Autodesk Fusion 360 part; units mm, degrees
note: some values were not read from the file. Set by a fixed rule: which sketch regions a step uses.
(part 4 of 14)
  spline S16 degree 5 poles (-6.8027, -18.1294) (-6.8027, -18.1295) (-6.8028, -18.1296) (-6.8029, -18.1298) (-6.803, -18.1302) (-6.8032, -18.1308) (-6.8035, -18.1315) (-6.8037, -18.1322) (-6.804, -18.133) (-6.8043, -18.1339) (-6.8047, -18.1349) (-6.8051, -18.136) (-6.8055, -18.1372) (-6.8059, -18.1384) (-6.8063, -18.1397) (-6.8068, -18.1411) (-6.8073, -18.1426) (-6.8078, -18.1442) (-6.8083, -18.1458) (-6.8089, -18.1475) (-6.8095, -18.1493) (-6.8101, -18.1512) (-6.8107, -18.1531) (-6.8113, -18.1552) (-6.812, -18.1572) (-6.8127, -18.1594) (-6.8134, -18.1617) (-6.8141, -18.164) (-6.8148, -18.1663) (-6.8155, -18.1688) (-6.8163, -18.1713) (-6.8171, -18.1739) (-6.8179, -18.1766) (-6.8187, -18.1793) (-6.8195, -18.1821) (-6.8203, -18.185) (-6.8212, -18.1879) (-6.822, -18.191) (-6.8229, -18.194) (-6.8238, -18.1972) (-6.8247, -18.2004) (-6.8256, -18.2037) (-6.8265, -18.207) (-6.8274, -18.2104) (-6.8284, -18.2139) (-6.8293, -18.2174) (-6.8303, -18.221) (-6.8312, -18.2247) (-6.8322, -18.2284) (-6.8332, -18.2322) (-6.8342, -18.236) (-6.8352, -18.2399) (-6.8362, -18.2439) (-6.8372, -18.2479) (-6.8382, -18.252) (-6.8392, -18.2561) (-6.8403, -18.2604) (-6.8413, -18.2646) (-6.8424, -18.269) (-6.8434, -18.2733) (-6.8445, -18.2778) (-6.8455, -18.2823) (-6.8466, -18.2868) (-6.8477, -18.2915) (-6.8487, -18.2961) (-6.8498, -18.3009) (-6.8509, -18.3057) (-6.852, -18.3105) (-6.8531, -18.3154) (-6.8542, -18.3203) (-6.8553, -18.3254) (-6.8564, -18.3304) (-6.8575, -18.3355) (-6.8586, -18.3407) (-6.8597, -18.3459) (-6.8608, -18.3512) (-6.8619, -18.3565) (-6.863, -18.3619) (-6.8641, -18.3674) (-6.8652, -18.3729) (-6.8663, -18.3784) (-6.8674, -18.384) (-6.8685, -18.3896) (-6.8696, -18.3953) (-6.8707, -18.4011) (-6.8718, -18.4069) (-6.8729, -18.4127) (-6.874, -18.4186) (-6.8751, -18.4246) (-6.8762, -18.4306) (-6.8773, -18.4366) (-6.8784, -18.4427) (-6.8795, -18.4489) (-6.8805, -18.4551) (-6.8816, -18.4613) (-6.8827, -18.4676) (-6.8838, -18.474) (-6.8849, -18.4804) (-6.8859, -18.4868) (-6.887, -18.4933) (-6.8881, -18.4998) (-6.8891, -18.5064) (-6.8902, -18.513) (-6.8912, -18.5197) (-6.8923, -18.5264) (-6.8933, -18.5332) (-6.8944, -18.54) (-6.8954, -18.5469) (-6.8964, -18.5538) (-6.8974, -18.5607) (-6.8985, -18.5677) (-6.8995, -18.5747) (-6.9005, -18.5818) (-6.9015, -18.5889) (-6.9025, -18.5961) (-6.9034, -18.6033) (-6.9044, -18.6106) (-6.9054, -18.6179) (-6.9064, -18.6252) (-6.9073, -18.6326) (-6.9083, -18.6401) (-6.9092, -18.6475) (-6.9102, -18.6551) (-6.9111, -18.6626) (-6.912, -18.6702) (-6.9129, -18.6779) (-6.9138, -18.6856) (-6.9147, -18.6933) (-6.9156, -18.7011) (-6.9165, -18.7089) (-6.9174, -18.7167) (-6.9182, -18.7246) (-6.9191, -18.7326) (-6.9199, -18.7405) (-6.9208, -18.7485) (-6.9216, -18.7566) (-6.9224, -18.7647) (-6.9232, -18.7728) (-6.924, -18.781) (-6.9248, -18.7892) (-6.9256, -18.7975) (-6.9264, -18.8058) (-6.9272, -18.8141) (-6.9279, -18.8225) (-6.9287, -18.8309) (-6.9294, -18.8394) (-6.9301, -18.8479) (-6.9308, -18.8564) (-6.9315, -18.8649) (-6.9322, -18.8736) (-6.9329, -18.8822) (-6.9336, -18.8909) (-6.9342, -18.8996) (-6.9349, -18.9084) (-6.9355, -18.9171) (-6.9361, -18.926) (-6.9367, -18.9348) (-6.9373, -18.9438) (-6.9379, -18.9527) (-6.9385, -18.9617) (-6.9391, -18.9707) (-6.9396, -18.9797) (-6.9402, -18.9888) (-6.9407, -18.9979) (-6.9412, -19.0071) (-6.9417, -19.0163) (-6.9422, -19.0255) (-6.9427, -19.0348) (-6.9431, -19.0441) (-6.9436, -19.0534) (-6.944, -19.0628) (-6.9445, -19.0722) (-6.9449, -19.0816) (-6.9453, -19.0911) (-6.9457, -19.1006) (-6.946, -19.1102) (-6.9464, -19.1198) (-6.9467, -19.1294) (-6.9471, -19.139) (-6.9474, -19.1487) (-6.9477, -19.1584) (-6.948, -19.1681) (-6.9483, -19.1779) (-6.9485, -19.1877) (-6.9488, -19.1976) (-6.949, -19.2075) (-6.9492, -19.2174) (-6.9495, -19.2273) (-6.9496, -19.2373) (-6.9498, -19.2473) (-6.95, -19.2574) (-6.9501, -19.2674) (-6.9503, -19.2775) (-6.9504, -19.2877) (-6.9505, -19.2979) (-6.9506, -19.3081) (-6.9507, -19.3183) (-6.9507, -19.3286) (-6.9508, -19.3389) (-6.9508, -19.3492) (-6.9508, -19.3595) (-6.9508, -19.3699) (-6.9508, -19.3804) (-6.9507, -19.3908) (-6.9507, -19.4013) (-6.9506, -19.4118) (-6.9505, -19.4224) (-6.9505, -19.4329) (-6.9503, -19.4435) (-6.9502, -19.4542) (-6.9501, -19.4648) (-6.9499, -19.4755) (-6.9497, -19.4863) (-6.9495, -19.497) (-6.9493, -19.5078) (-6.9491, -19.5186) (-6.9488, -19.5295) (-6.9486, -19.5403) (-6.9483, -19.5512) (-6.948, -19.5622) (-6.9477, -19.5731) (-6.9474, -19.5841) (-6.947, -19.5951) (-6.9467, -19.6062) (-6.9463, -19.6172) (-6.9459, -19.6283) (-6.9455, -19.6395) (-6.9451, -19.6506) (-6.9446, -19.6618) (-6.9441, -19.673) (-6.9437, -19.6843) (-6.9432, -19.6956) (-6.9426, -19.7068) (-6.9421, -19.7182) (-6.9416, -19.7295) (-6.941, -19.7409) (-6.9404, -19.7523) (-6.9398, -19.7637) (-6.9392, -19.7752) (-6.9385, -19.7867) (-6.9379, -19.7982) (-6.9373, -19.8074) (-6.9369, -19.8144) (-6.9366, -19.819) (-6.9365, -19.8213) knots 0 0 0 0 0 0 0.00416667 0.00833333 0.0125 0.01666667 0.02083333 0.025 0.02916667 0.03333333 0.0375 0.04166667 0.04583333 0.05 0.05416667 0.05833333 0.0625 0.06666667 0.07083333 0.075 0.07916667 0.08333333 0.0875 0.09166667 0.09583333 0.1 0.10416667 0.10833333 0.1125 0.11666667 0.12083333 0.125 0.12916667 0.13333333 0.1375 0.14166667 0.14583333 0.15 0.15416667 0.15833333 0.1625 0.16666667 0.17083333 0.175 0.17916667 0.18333333 0.1875 0.19166667 0.19583333 0.2 0.20416667 0.20833333 0.2125 0.21666667 0.22083333 0.225 0.22916667 0.23333333 0.2375 0.24166667 0.24583333 0.25 0.25416667 0.25833333 0.2625 0.26666667 0.27083333 0.275 0.27916667 0.28333333 0.2875 0.29166667 0.29583333 0.3 0.30416667 0.30833333 0.3125 0.31666667 0.32083333 0.325 0.32916667 0.33333333 0.3375 0.34166667 0.34583333 0.35 0.35416667 0.35833333 0.3625 0.36666667 0.37083333 0.375 0.37916667 0.38333333 0.3875 0.39166667 0.39583333 0.4 0.40416667 0.40833333 0.4125 0.41666667 0.42083333 0.425 0.42916667 0.43333333 0.4375 0.44166667 0.44583333 0.45 0.45416667 0.45833333 0.4625 0.46666667 0.47083333 0.475 0.47916667 0.48333333 0.4875 0.49166667 0.49583333 0.5 0.50416667 0.50833333 0.5125 0.51666667 0.52083333 0.525 0.52916667 0.53333333 0.5375 0.54166667 0.54583333 0.55 0.55416667 0.55833333 0.5625 0.56666667 0.57083333 0.575 0.57916667 0.58333333 0.5875 0.59166667 0.59583333 0.6 0.60416667 0.60833333 0.6125 0.61666667 0.62083333 0.625 0.62916667 0.63333333 0.6375 0.64166667 0.64583333 0.65 0.65416667 0.65833333 0.6625 0.66666667 0.67083333 0.675 0.67916667 0.68333333 0.6875 0.69166667 0.69583333 0.7 0.70416667 0.70833333 0.7125 0.71666667 0.72083333 0.725 0.72916667 0.73333333 0.7375 0.74166667 0.74583333 0.75 0.75416667 0.75833333 0.7625 0.76666667 0.77083333 0.775 0.77916667 0.78333333 0.7875 0.79166667 0.79583333 0.8 0.80416667 0.80833333 0.8125 0.81666667 0.82083333 0.825 0.82916667 0.83333333 0.8375 0.84166667 0.84583333 0.85 0.85416667 0.85833333 0.8625 0.86666667 0.87083333 0.875 0.87916667 0.88333333 0.8875 0.89166667 0.89583333 0.9 0.90416667 0.90833333 0.9125 0.91666667 0.92083333 0.925 0.92916667 0.93333333 0.9375 0.94166667 0.94583333 0.95 0.95416667 0.95833333 0.9625 0.96666667 0.97083333 0.975 0.97916667 0.98333333 0.9875 0.99166667 0.99583333 1 1 1 1 1 1
  arc A17 (-6.9365, -19.8213) -> (-6.039, -20.113) centre (0, 0) ccw
  spline S17 degree 5 poles (-6.039, -20.113) (-6.0375, -20.1112) (-6.0345, -20.1076) (-6.0301, -20.1022) (-6.0242, -20.0951) (-6.0169, -20.0861) (-6.0097, -20.0772) (-6.0024, -20.0683) (-5.9952, -20.0594) (-5.988, -20.0505) (-5.9809, -20.0417) (-5.9738, -20.0328) (-5.9667, -20.024) (-5.9596, -20.0151) (-5.9526, -20.0063) (-5.9456, -19.9975) (-5.9386, -19.9887) (-5.9317, -19.9799) (-5.9248, -19.9711) (-5.9179, -19.9624) (-5.9111, -19.9536) (-5.9042, -19.9449) (-5.8975, -19.9362) (-5.8907, -19.9274) (-5.884, -19.9187) (-5.8773, -19.9101) (-5.8706, -19.9014) (-5.864, -19.8927) (-5.8574, -19.8841) (-5.8508, -19.8755) (-5.8443, -19.8668) (-5.8378, -19.8582) (-5.8313, -19.8497) (-5.8248, -19.8411) (-5.8184, -19.8325) (-5.812, -19.824) (-5.8057, -19.8155) (-5.7994, -19.8069) (-5.7931, -19.7984) (-5.7868, -19.79) (-5.7806, -19.7815) (-5.7744, -19.773) (-5.7682, -19.7646) (-5.7621, -19.7562) (-5.7559, -19.7478) (-5.7499, -19.7394) (-5.7438, -19.731) (-5.7378, -19.7227) (-5.7318, -19.7143) (-5.7259, -19.706) (-5.7199, -19.6977) (-5.714, -19.6894) (-5.7082, -19.6811) (-5.7023, -19.6729) (-5.6965, -19.6646) (-5.6908, -19.6564) (-5.685, -19.6482) (-5.6793, -19.64) (-5.6736, -19.6319) (-5.668, -19.6237) (-5.6624, -19.6156) (-5.6568, -19.6075) (-5.6512, -19.5994) (-5.6457, -19.5913) (-5.6402, -19.5832) (-5.6348, -19.5752) (-5.6293, -19.5672) (-5.6239, -19.5592) (-5.6186, -19.5512) (-5.6132, -19.5432) (-5.6079, -19.5353) (-5.6026, -19.5274) (-5.5974, -19.5195) (-5.5922, -19.5116) (-5.587, -19.5037) (-5.5818, -19.4959) (-5.5767, -19.4881) (-5.5716, -19.4803) (-5.5666, -19.4725) (-5.5615, -19.4647) (-5.5565, -19.457) (-5.5516, -19.4493) (-5.5466, -19.4416) (-5.5417, -19.4339) (-5.5369, -19.4263) (-5.532, -19.4187) (-5.5272, -19.4111) (-5.5224, -19.4035) (-5.5177, -19.3959) (-5.513, -19.3884) (-5.5083, -19.3809) (-5.5036, -19.3734) (-5.499, -19.3659) (-5.4944, -19.3585) (-5.4899, -19.3511) (-5.4853, -19.3437) (-5.4808, -19.3363) (-5.4764, -19.329) (-5.4719, -19.3216) (-5.4675, -19.3144) (-5.4631, -19.3071) (-5.4588, -19.2998) (-5.4545, -19.2926) (-5.4502, -19.2854) (-5.4459, -19.2783) (-5.4417, -19.2711) (-5.4375, -19.264) (-5.4334, -19.2569) (-5.4293, -19.2499) (-5.4252, -19.2428) (-5.4211, -19.2358) (-5.4171, -19.2288) (-5.4131, -19.2219) (-5.4091, -19.215) (-5.4051, -19.2081) (-5.4012, -19.2012) (-5.3974, -19.1944) (-5.3935, -19.1876) (-5.3897, -19.1808) (-5.3859, -19.174) (-5.3822, -19.1673) (-5.3784, -19.1606) (-5.3747, -19.1539) (-5.3711, -19.1473) (-5.3674, -19.1407) (-5.3638, -19.1341) (-5.3603, -19.1276) (-5.3567, -19.1211) (-5.3532, -19.1146) (-5.3498, -19.1082) (-5.3463, -19.1017) (-5.3429, -19.0954) (-5.3395, -19.089) (-5.3362, -19.0827) (-5.3329, -19.0764) (-5.3296, -19.0701) (-5.3263, -19.0639) (-5.3231, -19.0577) (-5.3199, -19.0516) (-5.3167, -19.0455) (-5.3136, -19.0394) (-5.3105, -19.0333) (-5.3074, -19.0273) (-5.3044, -19.0213) (-5.3014, -19.0154) (-5.2984, -19.0095) (-5.2954, -19.0036) (-5.2925, -18.9978) (-5.2896, -18.9919) (-5.2868, -18.9862) (-5.2839, -18.9805) (-5.2812, -18.9748) (-5.2784, -18.9691) (-5.2757, -18.9635) (-5.273, -18.9579) (-5.2703, -18.9524) (-5.2676, -18.9469) (-5.265, -18.9414) (-5.2625, -18.936) (-5.2599, -18.9306) (-5.2574, -18.9253) (-5.2549, -18.92) (-5.2524, -18.9147) (-5.25, -18.9095) (-5.2476, -18.9043) (-5.2453, -18.8992) (-5.2429, -18.8941) (-5.2406, -18.8891) (-5.2383, -18.8841) (-5.2361, -18.8791) (-5.2339, -18.8742) (-5.2317, -18.8693) (-5.2296, -18.8645) (-5.2274, -18.8597) (-5.2253, -18.8549) (-5.2233, -18.8503) (-5.2213, -18.8456) (-5.2193, -18.841) (-5.2173, -18.8364) (-5.2154, -18.8319) (-5.2134, -18.8275) (-5.2116, -18.8231) (-5.2097, -18.8187) (-5.2079, -18.8144) (-5.2061, -18.8101) (-5.2044, -18.8059) (-5.2026, -18.8017) (-5.2009, -18.7976) (-5.1993, -18.7936) (-5.1976, -18.7895) (-5.196, -18.7856) (-5.1944, -18.7817) (-5.1929, -18.7778) (-5.1914, -18.774) (-5.1899, -18.7703) (-5.1884, -18.7666) (-5.187, -18.7629) (-5.1856, -18.7593) (-5.1842, -18.7558) (-5.1829, -18.7523) (-5.1816, -18.7489) (-5.1803, -18.7456) (-5.1791, -18.7423) (-5.1778, -18.739) (-5.1766, -18.7359) (-5.1755, -18.7327) (-5.1744, -18.7297) (-5.1732, -18.7267) (-5.1722, -18.7237) (-5.1711, -18.7209) (-5.1701, -18.718) (-5.1691, -18.7153) (-5.1682, -18.7126) (-5.1672, -18.71) (-5.1663, -18.7074) (-5.1655, -18.7049) (-5.1646, -18.7025) (-5.1638, -18.7002) (-5.163, -18.6979) (-5.1623, -18.6957) (-5.1615, -18.6935) (-5.1608, -18.6914) (-5.1602, -18.6894) (-5.1595, -18.6875) (-5.1589, -18.6856) (-5.1583, -18.6838) (-5.1578, -18.6821) (-5.1573, -18.6805) (-5.1568, -18.6789) (-5.1563, -18.6774) (-5.1558, -18.676) (-5.1554, -18.6747) (-5.155, -18.6734) (-5.1547, -18.6723) (-5.1543, -18.6712) (-5.154, -18.6702) (-5.1538, -18.6692) (-5.1535, -18.6684) (-5.1533, -18.6676) (-5.1531, -18.667) (-5.1529, -18.6664) (-5.1528, -18.666) (-5.1527, -18.6657) (-5.1527, -18.6656) (-5.1527, -18.6655) knots -1 -1 -1 -1 -1 -1 -0.99583333 -0.99166667 -0.9875 -0.98333333 -0.97916667 -0.975 -0.97083333 -0.96666667 -0.9625 -0.95833333 -0.95416667 -0.95 -0.94583333 -0.94166667 -0.9375 -0.93333333 -0.92916667 -0.925 -0.92083333 -0.91666667 -0.9125 -0.90833333 -0.90416667 -0.9 -0.89583333 -0.89166667 -0.8875 -0.88333333 -0.87916667 -0.875 -0.87083333 -0.86666667 -0.8625 -0.85833333 -0.85416667 -0.85 -0.84583333 -0.84166667 -0.8375 -0.83333333 -0.82916667 -0.825 -0.82083333 -0.81666667 -0.8125 -0.80833333 -0.80416667 -0.8 -0.79583333 -0.79166667 -0.7875 -0.78333333 -0.77916667 -0.775 -0.77083333 -0.76666667 -0.7625 -0.75833333 -0.75416667 -0.75 -0.74583333 -0.74166667 -0.7375 -0.73333333 -0.72916667 -0.725 -0.72083333 -0.71666667 -0.7125 -0.70833333 -0.70416667 -0.7 -0.69583333 -0.69166667 -0.6875 -0.68333333 -0.67916667 -0.675 -0.67083333 -0.66666667 -0.6625 -0.65833333 -0.65416667 -0.65 -0.64583333 -0.64166667 -0.6375 -0.63333333 -0.62916667 -0.625 -0.62083333 -0.61666667 -0.6125 -0.60833333 -0.60416667 -0.6 -0.59583333 -0.59166667 -0.5875 -0.58333333 -0.57916667 -0.575 -0.57083333 -0.56666667 -0.5625 -0.55833333 -0.55416667 -0.55 -0.54583333 -0.54166667 -0.5375 -0.53333333 -0.52916667 -0.525 -0.52083333 -0.51666667 -0.5125 -0.50833333 -0.50416667 -0.5 -0.49583333 -0.49166667 -0.4875 -0.48333333 -0.47916667 -0.475 -0.47083333 -0.46666667 -0.4625 -0.45833333 -0.45416667 -0.45 -0.44583333 -0.44166667 -0.4375 -0.43333333 -0.42916667 -0.425 -0.42083333 -0.41666667 -0.4125 -0.40833333 -0.40416667 -0.4 -0.39583333 -0.39166667 -0.3875 -0.38333333 -0.37916667 -0.375 -0.37083333 -0.36666667 -0.3625 -0.35833333 -0.35416667 -0.35 -0.34583333 -0.34166667 -0.3375 -0.33333333 -0.32916667 -0.325 -0.32083333 -0.31666667 -0.3125 -0.30833333 -0.30416667 -0.3 -0.29583333 -0.29166667 -0.2875 -0.28333333 -0.27916667 -0.275 -0.27083333 -0.26666667 -0.2625 -0.25833333 -0.25416667 -0.25 -0.24583333 -0.24166667 -0.2375 -0.23333333 -0.22916667 -0.225 -0.22083333 -0.21666667 -0.2125 -0.20833333 -0.20416667 -0.2 -0.19583333 -0.19166667 -0.1875 -0.18333333 -0.17916667 -0.175 -0.17083333 -0.16666667 -0.1625 -0.15833333 -0.15416667 -0.15 -0.14583333 -0.14166667 -0.1375 -0.13333333 -0.12916667 -0.125 -0.12083333 -0.11666667 -0.1125 -0.10833333 -0.10416667 -0.1 -0.09583333 -0.09166667 -0.0875 -0.08333333 -0.07916667 -0.075 -0.07083333 -0.06666667 -0.0625 -0.05833333 -0.05416667 -0.05 -0.04583333 -0.04166667 -0.0375 -0.03333333 -0.02916667 -0.025 -0.02083333 -0.01666667 -0.0125 -0.00833333 -0.00416667 0 0 0 0 0 0
  line L34 (-5.1527, -18.6655) -> (-5.1525, -18.6648)
  line L35 (-5.1525, -18.6648) -> (-4.9894, -18.074)
  arc A18 (-4.9894, -18.074) -> (-3.7599, -18.3692) centre (0, 0) ccw
  line L36 (-3.7599, -18.3692) -> (-3.8828, -18.9697)
  line L37 (-3.8828, -18.9697) -> (-3.8829, -18.9704)
  spline S18 degree 5 poles (-3.8829, -18.9704) (-3.8829, -18.9704) (-3.883, -18.9706) (-3.883, -18.9708) (-3.8831, -18.9712) (-3.8832, -18.9718) (-3.8833, -18.9725) (-3.8835, -18.9733) (-3.8836, -18.9742) (-3.8838, -18.9751) (-3.884, -18.9761) (-3.8842, -18.9773) (-3.8844, -18.9785) (-3.8846, -18.9798) (-3.8848, -18.9811) (-3.8851, -18.9826) (-3.8853, -18.9841) (-3.8856, -18.9858) (-3.8859, -18.9875) (-3.8862, -18.9892) (-3.8865, -18.9911) (-3.8868, -18.993) (-3.8871, -18.9951) (-3.8874, -18.9972) (-3.8877, -18.9993) (-3.888, -19.0016) (-3.8884, -19.0039) (-3.8887, -19.0063) (-3.889, -19.0088) (-3.8894, -19.0113) (-3.8898, -19.0139) (-3.8901, -19.0166) (-3.8905, -19.0194) (-3.8908, -19.0222) (-3.8912, -19.0251) (-3.8916, -19.0281) (-3.892, -19.0311) (-3.8923, -19.0342) (-3.8927, -19.0374) (-3.8931, -19.0406) (-3.8935, -19.0439) (-3.8939, -19.0473) (-3.8942, -19.0507) (-3.8946, -19.0542) (-3.895, -19.0578) (-3.8954, -19.0615) (-3.8958, -19.0652) (-3.8962, -19.0689) (-3.8965, -19.0727) (-3.8969, -19.0766) (-3.8973, -19.0806) (-3.8977, -19.0846) (-3.898, -19.0887) (-3.8984, -19.0928) (-3.8988, -19.097) (-3.8992, -19.1013) (-3.8995, -19.1056) (-3.8999, -19.11) (-3.9002, -19.1144) (-3.9006, -19.1189) (-3.9009, -19.1235) (-3.9013, -19.1281) (-3.9016, -19.1327) (-3.902, -19.1375) (-3.9023, -19.1423) (-3.9026, -19.1471) (-3.9029, -19.152) (-3.9032, -19.157) (-3.9035, -19.162) (-3.9039, -19.167) (-3.9041, -19.1721) (-3.9044, -19.1773) (-3.9047, -19.1825) (-3.905, -19.1878) (-3.9053, -19.1932) (-3.9055, -19.1985) (-3.9058, -19.204) (-3.906, -19.2095) (-3.9063, -19.215) (-3.9065, -19.2206) (-3.9067, -19.2263) (-3.9069, -19.232) (-3.9071, -19.2377) (-3.9073, -19.2435) (-3.9075, -19.2494) (-3.9077, -19.2553) (-3.9079, -19.2612) (-3.908, -19.2672) (-3.9082, -19.2733) (-3.9083, -19.2794) (-3.9085, -19.2855) (-3.9086, -19.2917) (-3.9087, -19.2979) (-3.9088, -19.3042) (-3.9089, -19.3106) (-3.909, -19.317) (-3.9091, -19.3234) (-3.9091, -19.3299) (-3.9092, -19.3364) (-3.9092, -19.343) (-3.9093, -19.3496) (-3.9093, -19.3563) (-3.9093, -19.363) (-3.9093, -19.3697) (-3.9093, -19.3765) (-3.9092, -19.3834) (-3.9092, -19.3903) (-3.9091, -19.3972) (-3.9091, -19.4042) (-3.909, -19.4112) (-3.9089, -19.4183) (-3.9088, -19.4254) (-3.9087, -19.4325) (-3.9085, -19.4397) (-3.9084, -19.447) (-3.9082, -19.4542) (-3.9081, -19.4616) (-3.9079, -19.4689) (-3.9077, -19.4763) (-3.9075, -19.4838) (-3.9073, -19.4913) (-3.907, -19.4988) (-3.9068, -19.5064) (-3.9065, -19.514) (-3.9062, -19.5216) (-3.9059, -19.5293) (-3.9056, -19.5371) (-3.9053, -19.5448) (-3.905, -19.5527) (-3.9046, -19.5605) (-3.9043, -19.5684) (-3.9039, -19.5763) (-3.9035, -19.5843) (-3.9031, -19.5923) (-3.9027, -19.6004) (-3.9022, -19.6085) (-3.9018, -19.6166) (-3.9013, -19.6248) (-3.9008, -19.633) (-3.9003, -19.6412) (-3.8998, -19.6495) (-3.8992, -19.6578) (-3.8987, -19.6661) (-3.8981, -19.6745) (-3.8975, -19.683) (-3.8969, -19.6914) (-3.8963, -19.6999) (-3.8957, -19.7084) (-3.8951, -19.717) (-3.8944, -19.7256) (-3.8937, -19.7343) (-3.893, -19.7429) (-3.8923, -19.7517) (-3.8916, -19.7604) (-3.8908, -19.7692) (-3.89, -19.778) (-3.8893, -19.7869) (-3.8885, -19.7958) (-3.8876, -19.8047) (-3.8868, -19.8136) (-3.886, -19.8226) (-3.8851, -19.8317) (-3.8842, -19.8407) (-3.8833, -19.8498) (-3.8824, -19.8589) (-3.8814, -19.8681) (-3.8805, -19.8773) (-3.8795, -19.8865) (-3.8785, -19.8958) (-3.8775, -19.9051) (-3.8765, -19.9144) (-3.8754, -19.9237) (-3.8743, -19.9331) (-3.8733, -19.9426) (-3.8722, -19.952) (-3.871, -19.9615) (-3.8699, -19.971) (-3.8687, -19.9806) (-3.8675, -19.9901) (-3.8663, -19.9997) (-3.8651, -20.0094) (-3.8639, -20.0191) (-3.8626, -20.0288) (-3.8614, -20.0385) (-3.8601, -20.0483) (-3.8588, -20.0581) (-3.8574, -20.0679) (-3.8561, -20.0777) (-3.8547, -20.0876) (-3.8533, -20.0975) (-3.8519, -20.1075) (-3.8505, -20.1175) (-3.849, -20.1275) (-3.8476, -20.1375) (-3.8461, -20.1476) (-3.8446, -20.1577) (-3.843, -20.1678) (-3.8415, -20.1779) (-3.8399, -20.1881) (-3.8383, -20.1983) (-3.8367, -20.2085) (-3.8351, -20.2188) (-3.8334, -20.2291) (-3.8318, -20.2394) (-3.8301, -20.2498) (-3.8284, -20.2601) (-3.8267, -20.2705) (-3.8249, -20.281) (-3.8231, -20.2914) (-3.8213, -20.3019) (-3.8195, -20.3124) (-3.8177, -20.323) (-3.8158, -20.3335) (-3.814, -20.3441) (-3.8121, -20.3547) (-3.8102, -20.3654) (-3.8082, -20.3761) (-3.8063, -20.3868) (-3.8043, -20.3975) (-3.8023, -20.4082) (-3.8003, -20.419) (-3.7982, -20.4298) (-3.7962, -20.4406) (-3.7941, -20.4515) (-3.792, -20.4624) (-3.7898, -20.4733) (-3.7877, -20.4842) (-3.7855, -20.4952) (-3.7833, -20.5061) (-3.7811, -20.5171) (-3.7789, -20.5282) (-3.7766, -20.5392) (-3.7743, -20.5503) (-3.772, -20.5614) (-3.7697, -20.5725) (-3.7674, -20.5837) (-3.765, -20.5948) (-3.7626, -20.606) (-3.7602, -20.6173) (-3.7578, -20.6285) (-3.7553, -20.6398) (-3.7533, -20.6488) (-3.7519, -20.6556) (-3.7508, -20.6601) (-3.7503, -20.6624) knots 0 0 0 0 0 0 0.00416667 0.00833333 0.0125 0.01666667 0.02083333 0.025 0.02916667 0.03333333 0.0375 0.04166667 0.04583333 0.05 0.05416667 0.05833333 0.0625 0.06666667 0.07083333 0.075 0.07916667 0.08333333 0.0875 0.09166667 0.09583333 0.1 0.10416667 0.10833333 0.1125 0.11666667 0.12083333 0.125 0.12916667 0.13333333 0.1375 0.14166667 0.14583333 0.15 0.15416667 0.15833333 0.1625 0.16666667 0.17083333 0.175 0.17916667 0.18333333 0.1875 0.19166667 0.19583333 0.2 0.20416667 0.20833333 0.2125 0.21666667 0.22083333 0.225 0.22916667 0.23333333 0.2375 0.24166667 0.24583333 0.25 0.25416667 0.25833333 0.2625 0.26666667 0.27083333 0.275 0.27916667 0.28333333 0.2875 0.29166667 0.29583333 0.3 0.30416667 0.30833333 0.3125 0.31666667 0.32083333 0.325 0.32916667 0.33333333 0.3375 0.34166667 0.34583333 0.35 0.35416667 0.35833333 0.3625 0.36666667 0.37083333 0.375 0.37916667 0.38333333 0.3875 0.39166667 0.39583333 0.4 0.40416667 0.40833333 0.4125 0.41666667 0.42083333 0.425 0.42916667 0.43333333 0.4375 0.44166667 0.44583333 0.45 0.45416667 0.45833333 0.4625 0.46666667 0.47083333 0.475 0.47916667 0.48333333 0.4875 0.49166667 0.49583333 0.5 0.50416667 0.50833333 0.5125 0.51666667 0.52083333 0.525 0.52916667 0.53333333 0.5375 0.54166667 0.54583333 0.55 0.55416667 0.55833333 0.5625 0.56666667 0.57083333 0.575 0.57916667 0.58333333 0.5875 0.59166667 0.59583333 0.6 0.60416667 0.60833333 0.6125 0.61666667 0.62083333 0.625 0.62916667 0.63333333 0.6375 0.64166667 0.64583333 0.65 0.65416667 0.65833333 0.6625 0.66666667 0.67083333 0.675 0.67916667 0.68333333 0.6875 0.69166667 0.69583333 0.7 0.70416667 0.70833333 0.7125 0.71666667 0.72083333 0.725 0.72916667 0.73333333 0.7375 0.74166667 0.74583333 0.75 0.75416667 0.75833333 0.7625 0.76666667 0.77083333 0.775 0.77916667 0.78333333 0.7875 0.79166667 0.79583333 0.8 0.80416667 0.80833333 0.8125 0.81666667 0.82083333 0.825 0.82916667 0.83333333 0.8375 0.84166667 0.84583333 0.85 0.85416667 0.85833333 0.8625 0.86666667 0.87083333 0.875 0.87916667 0.88333333 0.8875 0.89166667 0.89583333 0.9 0.90416667 0.90833333 0.9125 0.91666667 0.92083333 0.925 0.92916667 0.93333333 0.9375 0.94166667 0.94583333 0.95 0.95416667 0.95833333 0.9625 0.96666667 0.97083333 0.975 0.97916667 0.98333333 0.9875 0.99166667 0.99583333 1 1 1 1 1 1
  arc A19 (-3.7503, -20.6624) -> (-2.8182, -20.81) centre (0, 0) ccw
  spline S19 degree 5 poles (-2.8182, -20.81) (-2.8171, -20.808) (-2.8147, -20.804) (-2.8112, -20.798) (-2.8065, -20.7901) (-2.8007, -20.7801) (-2.7949, -20.7702) (-2.7892, -20.7602) (-2.7834, -20.7503) (-2.7777, -20.7404) (-2.772, -20.7305) (-2.7664, -20.7207) (-2.7608, -20.7108) (-2.7552, -20.701) (-2.7496, -20.6912) (-2.7441, -20.6814) (-2.7386, -20.6716) (-2.7331, -20.6618) (-2.7277, -20.6521) (-2.7222, -20.6424) (-2.7168, -20.6326) (-2.7115, -20.6229) (-2.7061, -20.6133) (-2.7008, -20.6036) (-2.6956, -20.594) (-2.6903, -20.5843) (-2.6851, -20.5747) (-2.6799, -20.5652) (-2.6747, -20.5556) (-2.6696, -20.546) (-2.6645, -20.5365) (-2.6594, -20.527) (-2.6543, -20.5175) (-2.6493, -20.508) (-2.6443, -20.4986) (-2.6393, -20.4891) (-2.6344, -20.4797) (-2.6295, -20.4703) (-2.6246, -20.4609) (-2.6197, -20.4516) (-2.6149, -20.4422) (-2.6101, -20.4329) (-2.6053, -20.4236) (-2.6006, -20.4143) (-2.5958, -20.4051) (-2.5912, -20.3958) (-2.5865, -20.3866) (-2.5818, -20.3774) (-2.5772, -20.3683) (-2.5727, -20.3591) (-2.5681, -20.35) (-2.5636, -20.3409) (-2.5591, -20.3318) (-2.5546, -20.3227) (-2.5502, -20.3137) (-2.5458, -20.3046) (-2.5414, -20.2956) (-2.537, -20.2867) (-2.5327, -20.2777) (-2.5284, -20.2688) (-2.5241, -20.2599) (-2.5199, -20.251) (-2.5156, -20.2421) (-2.5114, -20.2333) (-2.5073, -20.2245) (-2.5031, -20.2157) (-2.499, -20.2069) (-2.495, -20.1981) (-2.4909, -20.1894) (-2.4869, -20.1807) (-2.4829, -20.172) (-2.4789, -20.1634) (-2.475, -20.1548) (-2.471, -20.1462) (-2.4672, -20.1376) (-2.4633, -20.1291) (-2.4595, -20.1205) (-2.4557, -20.112) (-2.4519, -20.1036) (-2.4481, -20.0951) (-2.4444, -20.0867) (-2.4407, -20.0783) (-2.437, -20.0699) (-2.4334, -20.0616) (-2.4298, -20.0533) (-2.4262, -20.045) (-2.4226, -20.0367) (-2.4191, -20.0285) (-2.4156, -20.0203) (-2.4121, -20.0121) (-2.4086, -20.0039) (-2.4052, -19.9958) (-2.4018, -19.9877) (-2.3984, -19.9797) (-2.3951, -19.9716) (-2.3918, -19.9636) (-2.3885, -19.9556) (-2.3852, -19.9477) (-2.382, -19.9398) (-2.3788, -19.9319) (-2.3756, -19.924) (-2.3724, -19.9162) (-2.3693, -19.9084) (-2.3662, -19.9006) (-2.3631, -19.8929) (-2.3601, -19.8851) (-2.357, -19.8775) (-2.354, -19.8698) (-2.3511, -19.8622) (-2.3481, -19.8546) (-2.3452, -19.847) (-2.3423, -19.8395) (-2.3394, -19.832) (-2.3366, -19.8246) (-2.3338, -19.8171) (-2.331, -19.8098) (-2.3282, -19.8024) (-2.3255, -19.7951) (-2.3228, -19.7878) (-2.3201, -19.7805) (-2.3175, -19.7733) (-2.3148, -19.7661) (-2.3122, -19.7589) (-2.3097, -19.7518) (-2.3071, -19.7447) (-2.3046, -19.7377) (-2.3021, -19.7306) (-2.2996, -19.7237) (-2.2971, -19.7167) (-2.2947, -19.7098) (-2.2923, -19.7029) (-2.29, -19.6961) (-2.2876, -19.6893) (-2.2853, -19.6825) (-2.283, -19.6758) (-2.2807, -19.6691) (-2.2785, -19.6624) (-2.2763, -19.6558) (-2.2741, -19.6492) (-2.2719, -19.6427) (-2.2698, -19.6362) (-2.2676, -19.6297) (-2.2655, -19.6233) (-2.2635, -19.6169) (-2.2614, -19.6106) (-2.2594, -19.6043) (-2.2574, -19.598) (-2.2555, -19.5918) (-2.2535, -19.5856) (-2.2516, -19.5795) (-2.2497, -19.5734) (-2.2478, -19.5673) (-2.246, -19.5613) (-2.2442, -19.5553) (-2.2424, -19.5494) (-2.2406, -19.5435) (-2.2388, -19.5377) (-2.2371, -19.5319) (-2.2354, -19.5261) (-2.2337, -19.5204) (-2.2321, -19.5147) (-2.2305, -19.5091) (-2.2289, -19.5035) (-2.2273, -19.498) (-2.2257, -19.4925) (-2.2242, -19.4871) (-2.2227, -19.4817) (-2.2212, -19.4763) (-2.2197, -19.471) (-2.2183, -19.4658) (-2.2169, -19.4606) (-2.2155, -19.4554) (-2.2141, -19.4503) (-2.2128, -19.4452) (-2.2115, -19.4402) (-2.2102, -19.4353) (-2.2089, -19.4304) (-2.2076, -19.4255) (-2.2064, -19.4207) (-2.2052, -19.4159) (-2.204, -19.4112) (-2.2028, -19.4066) (-2.2017, -19.402) (-2.2006, -19.3974) (-2.1995, -19.393) (-2.1984, -19.3885) (-2.1973, -19.3841) (-2.1963, -19.3798) (-2.1953, -19.3755) (-2.1943, -19.3713) (-2.1933, -19.3671) (-2.1924, -19.363) (-2.1915, -19.359) (-2.1906, -19.355) (-2.1897, -19.3511) (-2.1888, -19.3472) (-2.188, -19.3434) (-2.1872, -19.3396) (-2.1864, -19.3359) (-2.1856, -19.3323) (-2.1848, -19.3287) (-2.1841, -19.3252) (-2.1834, -19.3217) (-2.1827, -19.3183) (-2.182, -19.315) (-2.1813, -19.3117) (-2.1807, -19.3085) (-2.1801, -19.3054) (-2.1795, -19.3023) (-2.1789, -19.2993) (-2.1783, -19.2964) (-2.1778, -19.2935) (-2.1772, -19.2907) (-2.1767, -19.288) (-2.1762, -19.2853) (-2.1758, -19.2827) (-2.1753, -19.2802) (-2.1749, -19.2777) (-2.1745, -19.2753) (-2.1741, -19.273) (-2.1737, -19.2708) (-2.1733, -19.2686) (-2.173, -19.2665) (-2.1726, -19.2645) (-2.1723, -19.2626) (-2.172, -19.2607) (-2.1718, -19.259) (-2.1715, -19.2573) (-2.1712, -19.2556) (-2.171, -19.2541) (-2.1708, -19.2526) (-2.1706, -19.2512) (-2.1704, -19.2499) (-2.1702, -19.2487) (-2.1701, -19.2476) (-2.1699, -19.2466) (-2.1698, -19.2456) (-2.1697, -19.2447) (-2.1696, -19.244) (-2.1695, -19.2433) (-2.1694, -19.2427) (-2.1694, -19.2423) (-2.1693, -19.242) (-2.1693, -19.2418) (-2.1693, -19.2418) knots -1 -1 -1 -1 -1 -1 -0.99583333 -0.99166667 -0.9875 -0.98333333 -0.97916667 -0.975 -0.97083333 -0.96666667 -0.9625 -0.95833333 -0.95416667 -0.95 -0.94583333 -0.94166667 -0.9375 -0.93333333 -0.92916667 -0.925 -0.92083333 -0.91666667 -0.9125 -0.90833333 -0.90416667 -0.9 -0.89583333 -0.89166667 -0.8875 -0.88333333 -0.87916667 -0.875 -0.87083333 -0.86666667 -0.8625 -0.85833333 -0.85416667 -0.85 -0.84583333 -0.84166667 -0.8375 -0.83333333 -0.82916667 -0.825 -0.82083333 -0.81666667 -0.8125 -0.80833333 -0.80416667 -0.8 -0.79583333 -0.79166667 -0.7875 -0.78333333 -0.77916667 -0.775 -0.77083333 -0.76666667 -0.7625 -0.75833333 -0.75416667 -0.75 -0.74583333 -0.74166667 -0.7375 -0.73333333 -0.72916667 -0.725 -0.72083333 -0.71666667 -0.7125 -0.70833333 -0.70416667 -0.7 -0.69583333 -0.69166667 -0.6875 -0.68333333 -0.67916667 -0.675 -0.67083333 -0.66666667 -0.6625 -0.65833333 -0.65416667 -0.65 -0.64583333 -0.64166667 -0.6375 -0.63333333 -0.62916667 -0.625 -0.62083333 -0.61666667 -0.6125 -0.60833333 -0.60416667 -0.6 -0.59583333 -0.59166667 -0.5875 -0.58333333 -0.57916667 -0.575 -0.57083333 -0.56666667 -0.5625 -0.55833333 -0.55416667 -0.55 -0.54583333 -0.54166667 -0.5375 -0.53333333 -0.52916667 -0.525 -0.52083333 -0.51666667 -0.5125 -0.50833333 -0.50416667 -0.5 -0.49583333 -0.49166667 -0.4875 -0.48333333 -0.47916667 -0.475 -0.47083333 -0.46666667 -0.4625 -0.45833333 -0.45416667 -0.45 -0.44583333 -0.44166667 -0.4375 -0.43333333 -0.42916667 -0.425 -0.42083333 -0.41666667 -0.4125 -0.40833333 -0.40416667 -0.4 -0.39583333 -0.39166667 -0.3875 -0.38333333 -0.37916667 -0.375 -0.37083333 -0.36666667 -0.3625 -0.35833333 -0.35416667 -0.35 -0.34583333 -0.34166667 -0.3375 -0.33333333 -0.32916667 -0.325 -0.32083333 -0.31666667 -0.3125 -0.30833333 -0.30416667 -0.3 -0.29583333 -0.29166667 -0.2875 -0.28333333 -0.27916667 -0.275 -0.27083333 -0.26666667 -0.2625 -0.25833333 -0.25416667 -0.25 -0.24583333 -0.24166667 -0.2375 -0.23333333 -0.22916667 -0.225 -0.22083333 -0.21666667 -0.2125 -0.20833333 -0.20416667 -0.2 -0.19583333 -0.19166667 -0.1875 -0.18333333 -0.17916667 -0.175 -0.17083333 -0.16666667 -0.1625 -0.15833333 -0.15416667 -0.15 -0.14583333 -0.14166667 -0.1375 -0.13333333 -0.12916667 -0.125 -0.12083333 -0.11666667 -0.1125 -0.10833333 -0.10416667 -0.1 -0.09583333 -0.09166667 -0.0875 -0.08333333 -0.07916667 -0.075 -0.07083333 -0.06666667 -0.0625 -0.05833333 -0.05416667 -0.05 -0.04583333 -0.04166667 -0.0375 -0.03333333 -0.02916667 -0.025 -0.02083333 -0.01666667 -0.0125 -0.00833333 -0.00416667 0 0 0 0 0 0
  line L38 (-2.1693, -19.2418) -> (-2.1692, -19.2411)
  line L39 (-2.1692, -19.2411) -> (-2.1005, -18.632)
  arc A20 (-2.1005, -18.632) -> (-0.84, -18.7312) centre (0, 0) ccw
  line L40 (-0.84, -18.7312) -> (-0.8675, -19.3435)
  line L41 (-0.8675, -19.3435) -> (-0.8675, -19.3442)
  spline S20 degree 5 poles (-0.8675, -19.3442) (-0.8675, -19.3443) (-0.8675, -19.3445) (-0.8675, -19.3447) (-0.8675, -19.3451) (-0.8675, -19.3457) (-0.8676, -19.3464) (-0.8676, -19.3472) (-0.8676, -19.3481) (-0.8676, -19.3491) (-0.8676, -19.3501) (-0.8677, -19.3512) (-0.8677, -19.3525) (-0.8677, -19.3538) (-0.8677, -19.3552) (-0.8677, -19.3567) (-0.8677, -19.3582) (-0.8677, -19.3599) (-0.8677, -19.3616) (-0.8677, -19.3634) (-0.8677, -19.3653) (-0.8677, -19.3672) (-0.8677, -19.3693) (-0.8677, -19.3714) (-0.8677, -19.3736) (-0.8677, -19.3759) (-0.8676, -19.3782) (-0.8676, -19.3806) (-0.8675, -19.3831) (-0.8675, -19.3857) (-0.8674, -19.3883) (-0.8674, -19.391) (-0.8673, -19.3938) (-0.8672, -19.3967) (-0.8671, -19.3996) (-0.867, -19.4026) (-0.8669, -19.4056) (-0.8668, -19.4087) (-0.8667, -19.4119) (-0.8666, -19.4152) (-0.8664, -19.4185) (-0.8663, -19.4219) (-0.8661, -19.4254) (-0.8659, -19.4289) (-0.8658, -19.4325) (-0.8656, -19.4361) (-0.8654, -19.4399) (-0.8652, -19.4436) (-0.8649, -19.4475) (-0.8647, -19.4514) (-0.8645, -19.4553) (-0.8642, -19.4594) (-0.8639, -19.4635) (-0.8636, -19.4676) (-0.8634, -19.4718) (-0.8631, -19.4761) (-0.8627, -19.4804) (-0.8624, -19.4848) (-0.8621, -19.4892) (-0.8617, -19.4937) (-0.8613, -19.4983) (-0.861, -19.5029) (-0.8606, -19.5075) (-0.8602, -19.5123) (-0.8597, -19.517) (-0.8593, -19.5219) (-0.8588, -19.5268) (-0.8584, -19.5317) (-0.8579, -19.5367) (-0.8574, -19.5417) (-0.8569, -19.5468) (-0.8564, -19.552) (-0.8558, -19.5572) (-0.8553, -19.5625) (-0.8547, -19.5678) (-0.8541, -19.5731) (-0.8535, -19.5785) (-0.8529, -19.584) (-0.8523, -19.5895) (-0.8516, -19.5951) (-0.851, -19.6007) (-0.8503, -19.6064) (-0.8496, -19.6121) (-0.8489, -19.6178) (-0.8482, -19.6236) (-0.8474, -19.6295) (-0.8467, -19.6354) (-0.8459, -19.6414) (-0.8451, -19.6474) (-0.8443, -19.6534) (-0.8434, -19.6595) (-0.8426, -19.6656) (-0.8417, -19.6718) (-0.8409, -19.678) (-0.84, -19.6843) (-0.839, -19.6906) (-0.8381, -19.697) (-0.8371, -19.7034) (-0.8362, -19.7099) (-0.8352, -19.7164) (-0.8342, -19.7229) (-0.8332, -19.7295) (-0.8321, -19.7361) (-0.831, -19.7428) (-0.83, -19.7495) (-0.8289, -19.7563) (-0.8277, -19.7631) (-0.8266, -19.7699) (-0.8255, -19.7768) (-0.8243, -19.7837) (-0.8231, -19.7907) (-0.8219, -19.7977) (-0.8206, -19.8047) (-0.8194, -19.8118) (-0.8181, -19.8189) (-0.8168, -19.8261) (-0.8155, -19.8333) (-0.8142, -19.8406) (-0.8128, -19.8478) (-0.8115, -19.8552) (-0.8101, -19.8625) (-0.8086, -19.8699) (-0.8072, -19.8774) (-0.8058, -19.8849) (-0.8043, -19.8924) (-0.8028, -19.8999) (-0.8013, -19.9075) (-0.7998, -19.9151) (-0.7982, -19.9228) (-0.7966, -19.9305) (-0.795, -19.9382) (-0.7934, -19.946) (-0.7918, -19.9538) (-0.7901, -19.9617) (-0.7884, -19.9696) (-0.7867, -19.9775) (-0.785, -19.9854) (-0.7833, -19.9934) (-0.7815, -20.0015) (-0.7797, -20.0095) (-0.7779, -20.0176) (-0.7761, -20.0257) (-0.7742, -20.0339) (-0.7724, -20.0421) (-0.7705, -20.0503) (-0.7686, -20.0586) (-0.7666, -20.0669) (-0.7647, -20.0752) (-0.7627, -20.0836) (-0.7607, -20.092) (-0.7586, -20.1004) (-0.7566, -20.1089) (-0.7545, -20.1174) (-0.7524, -20.1259) (-0.7503, -20.1345) (-0.7482, -20.1431) (-0.746, -20.1517) (-0.7439, -20.1603) (-0.7416, -20.169) (-0.7394, -20.1777) (-0.7372, -20.1865) (-0.7349, -20.1953) (-0.7326, -20.2041) (-0.7303, -20.2129) (-0.728, -20.2218) (-0.7256, -20.2307) (-0.7232, -20.2396) (-0.7208, -20.2486) (-0.7184, -20.2576) (-0.7159, -20.2666) (-0.7134, -20.2756) (-0.7109, -20.2847) (-0.7084, -20.2938) (-0.7059, -20.3029) (-0.7033, -20.3121) (-0.7007, -20.3213) (-0.6981, -20.3305) (-0.6954, -20.3398) (-0.6928, -20.349) (-0.6901, -20.3583) (-0.6874, -20.3677) (-0.6847, -20.377) (-0.6819, -20.3864) (-0.6791, -20.3958) (-0.6763, -20.4053) (-0.6735, -20.4148) (-0.6706, -20.4243) (-0.6678, -20.4338) (-0.6649, -20.4433) (-0.6619, -20.4529) (-0.659, -20.4625) (-0.656, -20.4721) (-0.653, -20.4818) (-0.65, -20.4915) (-0.6469, -20.5012) (-0.6439, -20.5109) (-0.6408, -20.5207) (-0.6377, -20.5304) (-0.6345, -20.5402) (-0.6314, -20.5501) (-0.6282, -20.5599) (-0.625, -20.5698) (-0.6217, -20.5797) (-0.6185, -20.5897) (-0.6152, -20.5996) (-0.6119, -20.6096) (-0.6085, -20.6196) (-0.6052, -20.6296) (-0.6018, -20.6397) (-0.5984, -20.6498) (-0.5949, -20.6598) (-0.5915, -20.67) (-0.588, -20.6801) (-0.5845, -20.6903) (-0.581, -20.7005) (-0.5774, -20.7107) (-0.5738, -20.7209) (-0.5702, -20.7312) (-0.5666, -20.7415) (-0.5629, -20.7518) (-0.5592, -20.7621) (-0.5555, -20.7725) (-0.5518, -20.7828) (-0.548, -20.7932) (-0.5443, -20.8036) (-0.5405, -20.8141) (-0.5366, -20.8245) (-0.5328, -20.835) (-0.5289, -20.8455) (-0.525, -20.856) (-0.521, -20.8666) (-0.5171, -20.8771) (-0.5131, -20.8877) (-0.5091, -20.8983) (-0.5051, -20.909) (-0.501, -20.9196) (-0.4969, -20.9303) (-0.4928, -20.941) (-0.4887, -20.9517) (-0.4845, -20.9624) (-0.4803, -20.9731) (-0.4769, -20.9818) (-0.4744, -20.9882) (-0.4727, -20.9925) (-0.4719, -20.9947) knots 0 0 0 0 0 0 0.00416667 0.00833333 0.0125 0.01666667 0.02083333 0.025 0.02916667 0.03333333 0.0375 0.04166667 0.04583333 0.05 0.05416667 0.05833333 0.0625 0.06666667 0.07083333 0.075 0.07916667 0.08333333 0.0875 0.09166667 0.09583333 0.1 0.10416667 0.10833333 0.1125 0.11666667 0.12083333 0.125 0.12916667 0.13333333 0.1375 0.14166667 0.14583333 0.15 0.15416667 0.15833333 0.1625 0.16666667 0.17083333 0.175 0.17916667 0.18333333 0.1875 0.19166667 0.19583333 0.2 0.20416667 0.20833333 0.2125 0.21666667 0.22083333 0.225 0.22916667 0.23333333 0.2375 0.24166667 0.24583333 0.25 0.25416667 0.25833333 0.2625 0.26666667 0.27083333 0.275 0.27916667 0.28333333 0.2875 0.29166667 0.29583333 0.3 0.30416667 0.30833333 0.3125 0.31666667 0.32083333 0.325 0.32916667 0.33333333 0.3375 0.34166667 0.34583333 0.35 0.35416667 0.35833333 0.3625 0.36666667 0.37083333 0.375 0.37916667 0.38333333 0.3875 0.39166667 0.39583333 0.4 0.40416667 0.40833333 0.4125 0.41666667 0.42083333 0.425 0.42916667 0.43333333 0.4375 0.44166667 0.44583333 0.45 0.45416667 0.45833333 0.4625 0.46666667 0.47083333 0.475 0.47916667 0.48333333 0.4875 0.49166667 0.49583333 0.5 0.50416667 0.50833333 0.5125 0.51666667 0.52083333 0.525 0.52916667 0.53333333 0.5375 0.54166667 0.54583333 0.55 0.55416667 0.55833333 0.5625 0.56666667 0.57083333 0.575 0.57916667 0.58333333 0.5875 0.59166667 0.59583333 0.6 0.60416667 0.60833333 0.6125 0.61666667 0.62083333 0.625 0.62916667 0.63333333 0.6375 0.64166667 0.64583333 0.65 0.65416667 0.65833333 0.6625 0.66666667 0.67083333 0.675 0.67916667 0.68333333 0.6875 0.69166667 0.69583333 0.7 0.70416667 0.70833333 0.7125 0.71666667 0.72083333 0.725 0.72916667 0.73333333 0.7375 0.74166667 0.74583333 0.75 0.75416667 0.75833333 0.7625 0.76666667 0.77083333 0.775 0.77916667 0.78333333 0.7875 0.79166667 0.79583333 0.8 0.80416667 0.80833333 0.8125 0.81666667 0.82083333 0.825 0.82916667 0.83333333 0.8375 0.84166667 0.84583333 0.85 0.85416667 0.85833333 0.8625 0.86666667 0.87083333 0.875 0.87916667 0.88333333 0.8875 0.89166667 0.89583333 0.9 0.90416667 0.90833333 0.9125 0.91666667 0.92083333 0.925 0.92916667 0.93333333 0.9375 0.94166667 0.94583333 0.95 0.95416667 0.95833333 0.9625 0.96666667 0.97083333 0.975 0.97916667 0.98333333 0.9875 0.99166667 0.99583333 1 1 1 1 1 1
  arc A21 (-0.4719, -20.9947) -> (0.4719, -20.9947) centre (0, 0) ccw
  spline S21 degree 5 poles (0.4719, -20.9947) (0.4727, -20.9925) (0.4744, -20.9882) (0.4769, -20.9818) (0.4803, -20.9731) (0.4845, -20.9624) (0.4887, -20.9517) (0.4928, -20.941) (0.4969, -20.9303) (0.501, -20.9196) (0.5051, -20.909) (0.5091, -20.8983) (0.5131, -20.8877) (0.5171, -20.8771) (0.521, -20.8666) (0.525, -20.856) (0.5289, -20.8455) (0.5328, -20.835) (0.5366, -20.8245) (0.5405, -20.8141) (0.5443, -20.8036) (0.548, -20.7932) (0.5518, -20.7828) (0.5555, -20.7725) (0.5592, -20.7621) (0.5629, -20.7518) (0.5666, -20.7415) (0.5702, -20.7312) (0.5738, -20.7209) (0.5774, -20.7107) (0.581, -20.7005) (0.5845, -20.6903) (0.588, -20.6801) (0.5915, -20.67) (0.5949, -20.6598) (0.5984, -20.6498) (0.6018, -20.6397) (0.6052, -20.6296) (0.6085, -20.6196) (0.6119, -20.6096) (0.6152, -20.5996) (0.6185, -20.5897) (0.6217, -20.5797) (0.625, -20.5698) (0.6282, -20.5599) (0.6314, -20.5501) (0.6345, -20.5402) (0.6377, -20.5304) (0.6408, -20.5207) (0.6439, -20.5109) (0.6469, -20.5012) (0.65, -20.4915) (0.653, -20.4818) (0.656, -20.4721) (0.659, -20.4625) (0.6619, -20.4529) (0.6649, -20.4433) (0.6678, -20.4338) (0.6706, -20.4243) (0.6735, -20.4148) (0.6763, -20.4053) (0.6791, -20.3958) (0.6819, -20.3864) (0.6847, -20.377) (0.6874, -20.3677) (0.6901, -20.3583) (0.6928, -20.349) (0.6954, -20.3398) (0.6981, -20.3305) (0.7007, -20.3213) (0.7033, -20.3121) (0.7059, -20.3029) (0.7084, -20.2938) (0.7109, -20.2847) (0.7134, -20.2756) (0.7159, -20.2666) (0.7184, -20.2576) (0.7208, -20.2486) (0.7232, -20.2396) (0.7256, -20.2307) (0.728, -20.2218) (0.7303, -20.2129) (0.7326, -20.2041) (0.7349, -20.1953) (0.7372, -20.1865) (0.7394, -20.1777) (0.7416, -20.169) (0.7439, -20.1603) (0.746, -20.1517) (0.7482, -20.1431) (0.7503, -20.1345) (0.7524, -20.1259) (0.7545, -20.1174) (0.7566, -20.1089) (0.7586, -20.1004) (0.7607, -20.092) (0.7627, -20.0836) (0.7647, -20.0752) (0.7666, -20.0669) (0.7686, -20.0586) (0.7705, -20.0503) (0.7724, -20.0421) (0.7742, -20.0339) (0.7761, -20.0257) (0.7779, -20.0176) (0.7797, -20.0095) (0.7815, -20.0015) (0.7833, -19.9934) (0.785, -19.9854) (0.7867, -19.9775) (0.7884, -19.9696) (0.7901, -19.9617) (0.7918, -19.9538) (0.7934, -19.946) (0.795, -19.9382) (0.7966, -19.9305) (0.7982, -19.9228) (0.7998, -19.9151) (0.8013, -19.9075) (0.8028, -19.8999) (0.8043, -19.8924) (0.8058, -19.8849) (0.8072, -19.8774) (0.8086, -19.8699) (0.8101, -19.8625) (0.8115, -19.8552) (0.8128, -19.8478) (0.8142, -19.8406) (0.8155, -19.8333) (0.8168, -19.8261) (0.8181, -19.8189) (0.8194, -19.8118) (0.8206, -19.8047) (0.8219, -19.7977) (0.8231, -19.7907) (0.8243, -19.7837) (0.8255, -19.7768) (0.8266, -19.7699) (0.8277, -19.7631) (0.8289, -19.7563) (0.83, -19.7495) (0.831, -19.7428) (0.8321, -19.7361) (0.8332, -19.7295) (0.8342, -19.7229) (0.8352, -19.7164) (0.8362, -19.7099) (0.8371, -19.7034) (0.8381, -19.697) (0.839, -19.6906) (0.84, -19.6843) (0.8409, -19.678) (0.8417, -19.6718) (0.8426, -19.6656) (0.8434, -19.6595) (0.8443, -19.6534) (0.8451, -19.6474) (0.8459, -19.6414) (0.8467, -19.6354) (0.8474, -19.6295) (0.8482, -19.6236) (0.8489, -19.6178) (0.8496, -19.6121) (0.8503, -19.6064) (0.851, -19.6007) (0.8516, -19.5951) (0.8523, -19.5895) (0.8529, -19.584) (0.8535, -19.5785) (0.8541, -19.5731) (0.8547, -19.5678) (0.8553, -19.5625) (0.8558, -19.5572) (0.8564, -19.552) (0.8569, -19.5468) (0.8574, -19.5417) (0.8579, -19.5367) (0.8584, -19.5317) (0.8588, -19.5268) (0.8593, -19.5219) (0.8597, -19.517) (0.8602, -19.5123) (0.8606, -19.5075) (0.861, -19.5029) (0.8613, -19.4983) (0.8617, -19.4937) (0.8621, -19.4892) (0.8624, -19.4848) (0.8627, -19.4804) (0.8631, -19.4761) (0.8634, -19.4718) (0.8636, -19.4676) (0.8639, -19.4635) (0.8642, -19.4594) (0.8645, -19.4553) (0.8647, -19.4514) (0.8649, -19.4475) (0.8652, -19.4436) (0.8654, -19.4399) (0.8656, -19.4361) (0.8658, -19.4325) (0.8659, -19.4289) (0.8661, -19.4254) (0.8663, -19.4219) (0.8664, -19.4185) (0.8666, -19.4152) (0.8667, -19.4119) (0.8668, -19.4087) (0.8669, -19.4056) (0.867, -19.4026) (0.8671, -19.3996) (0.8672, -19.3967) (0.8673, -19.3938) (0.8674, -19.391) (0.8674, -19.3883) (0.8675, -19.3857) (0.8675, -19.3831) (0.8676, -19.3806) (0.8676, -19.3782) (0.8677, -19.3759) (0.8677, -19.3736) (0.8677, -19.3714) (0.8677, -19.3693) (0.8677, -19.3672) (0.8677, -19.3653) (0.8677, -19.3634) (0.8677, -19.3616) (0.8677, -19.3599) (0.8677, -19.3582) (0.8677, -19.3567) (0.8677, -19.3552) (0.8677, -19.3538) (0.8677, -19.3525) (0.8677, -19.3512) (0.8676, -19.3501) (0.8676, -19.3491) (0.8676, -19.3481) (0.8676, -19.3472) (0.8676, -19.3464) (0.8675, -19.3457) (0.8675, -19.3451) (0.8675, -19.3447) (0.8675, -19.3445) (0.8675, -19.3443) (0.8675, -19.3442) knots -1 -1 -1 -1 -1 -1 -0.99583333 -0.99166667 -0.9875 -0.98333333 -0.97916667 -0.975 -0.97083333 -0.96666667 -0.9625 -0.95833333 -0.95416667 -0.95 -0.94583333 -0.94166667 -0.9375 -0.93333333 -0.92916667 -0.925 -0.92083333 -0.91666667 -0.9125 -0.90833333 -0.90416667 -0.9 -0.89583333 -0.89166667 -0.8875 -0.88333333 -0.87916667 -0.875 -0.87083333 -0.86666667 -0.8625 -0.85833333 -0.85416667 -0.85 -0.84583333 -0.84166667 -0.8375 -0.83333333 -0.82916667 -0.825 -0.82083333 -0.81666667 -0.8125 -0.80833333 -0.80416667 -0.8 -0.79583333 -0.79166667 -0.7875 -0.78333333 -0.77916667 -0.775 -0.77083333 -0.76666667 -0.7625 -0.75833333 -0.75416667 -0.75 -0.74583333 -0.74166667 -0.7375 -0.73333333 -0.72916667 -0.725 -0.72083333 -0.71666667 -0.7125 -0.70833333 -0.70416667 -0.7 -0.69583333 -0.69166667 -0.6875 -0.68333333 -0.67916667 -0.675 -0.67083333 -0.66666667 -0.6625 -0.65833333 -0.65416667 -0.65 -0.64583333 -0.64166667 -0.6375 -0.63333333 -0.62916667 -0.625 -0.62083333 -0.61666667 -0.6125 -0.60833333 -0.60416667 -0.6 -0.59583333 -0.59166667 -0.5875 -0.58333333 -0.57916667 -0.575 -0.57083333 -0.56666667 -0.5625 -0.55833333 -0.55416667 -0.55 -0.54583333 -0.54166667 -0.5375 -0.53333333 -0.52916667 -0.525 -0.52083333 -0.51666667 -0.5125 -0.50833333 -0.50416667 -0.5 -0.49583333 -0.49166667 -0.4875 -0.48333333 -0.47916667 -0.475 -0.47083333 -0.46666667 -0.4625 -0.45833333 -0.45416667 -0.45 -0.44583333 -0.44166667 -0.4375 -0.43333333 -0.42916667 -0.425 -0.42083333 -0.41666667 -0.4125 -0.40833333 -0.40416667 -0.4 -0.39583333 -0.39166667 -0.3875 -0.38333333 -0.37916667 -0.375 -0.37083333 -0.36666667 -0.3625 -0.35833333 -0.35416667 -0.35 -0.34583333 -0.34166667 -0.3375 -0.33333333 -0.32916667 -0.325 -0.32083333 -0.31666667 -0.3125 -0.30833333 -0.30416667 -0.3 -0.29583333 -0.29166667 -0.2875 -0.28333333 -0.27916667 -0.275 -0.27083333 -0.26666667 -0.2625 -0.25833333 -0.25416667 -0.25 -0.24583333 -0.24166667 -0.2375 -0.23333333 -0.22916667 -0.225 -0.22083333 -0.21666667 -0.2125 -0.20833333 -0.20416667 -0.2 -0.19583333 -0.19166667 -0.1875 -0.18333333 -0.17916667 -0.175 -0.17083333 -0.16666667 -0.1625 -0.15833333 -0.15416667 -0.15 -0.14583333 -0.14166667 -0.1375 -0.13333333 -0.12916667 -0.125 -0.12083333 -0.11666667 -0.1125 -0.10833333 -0.10416667 -0.1 -0.09583333 -0.09166667 -0.0875 -0.08333333 -0.07916667 -0.075 -0.07083333 -0.06666667 -0.0625 -0.05833333 -0.05416667 -0.05 -0.04583333 -0.04166667 -0.0375 -0.03333333 -0.02916667 -0.025 -0.02083333 -0.01666667 -0.0125 -0.00833333 -0.00416667 0 0 0 0 0 0
  line L42 (0.8675, -19.3442) -> (0.8675, -19.3435)
  line L43 (0.8675, -19.3435) -> (0.84, -18.7312)
  arc A22 (0.84, -18.7312) -> (2.1005, -18.632) centre (0, 0) ccw
  line L44 (2.1005, -18.632) -> (2.1692, -19.2411)
  line L45 (2.1692, -19.2411) -> (2.1693, -19.2418)